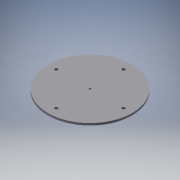
# Autodesk Inventor part: Keep Out RSX Deck
Saved by Autodesk Inventor 2016 (Build 200138000, 138)
## iProperties
Created: 2016-10-29
Part Number: Keep Out RSX Deck
Material: Generic
Document SubType Name: Modeling
Designer: eschr_000
Density: 1 g/cm^3
Appearance: Default
Author: eschr_000
Autodesk Inventor part; units mm, degrees
ref_plane "YZ Plane" through (0, 0, 0) normal (1, 0, 0) x (0, 1, 0)
ref_plane "XZ Plane" through (0, 0, 0) normal (0, 1, 0) x (-1, 0, 0)
ref_plane "XY Plane" through (0, 0, 0) normal (0, 0, 1) x (1, 0, 0)
sketch "Sketch1" plane through (0, 0, 0) normal (0, 1, 0) x (-1, 0, 0)
  circle A0 centre (0, 0) radius 127
  dimension "d0" = 254
  constraints: 1 centre point, 1 coincident
  measures "d0" diameter of A0
extrude "Extrusion1" add sketch "Sketch1" along normal blind 6.35
sketch "Sketch2" plane through (0, 6.35, 0) normal (0, 1, 0) x (1, 0, 0)
  point P0 (0, 0)
  point P1 (0, 0)
  constraints: 1 coincident
hole "Hole1" at (0, 6.35, 0) direction (0, -1, 0) diameter 6.0452 end through all
sketch "Sketch3" plane through (0, 6.35, 0) normal (0, 1, 0) x (1, 0, 0)
  circle A0 centre (0, 0) radius 3.0226 projected
  circle A1 centre (0, 0) radius 101.6
  point P0 (-101.6, 0)
  point P1 (0, -101.6)
  point P2 (0, 101.6)
  point P3 (101.6, 0)
  dimension "d10" = 203.2
  constraints: 4 point on circle, 1 centre point, 1 coincident
  measures "d10" diameter of A1
hole "Hole2" at (-101.6, 6.35, 0) at (0, 6.35, 101.6) at (0, 6.35, -101.6) at (101.6, 6.35, 0) direction (0, -1, 0) diameter 9.8044 end through all
body "Solid1"
